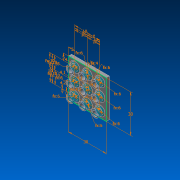
# Autodesk Inventor part: collet test
Saved by Autodesk Inventor 2015 (Build 190159000, 159)
## iProperties
Created: 2017-03-17
Part Number: collet test
Material: Generic
Document SubType Name: Modeling
Designer: ZigZagJoe
Density: 1 g/cm^3
Appearance: Default
Author: ZigZagJoe
Autodesk Inventor part; units mm, degrees
ref_plane "YZ Plane" through (0, 0, 0) normal (1, 0, 0) x (0, 1, 0)
ref_plane "XZ Plane" through (0, 0, 0) normal (0, 1, 0) x (-1, 0, 0)
ref_plane "XY Plane" through (0, 0, 0) normal (0, 0, 1) x (1, 0, 0)
sketch "Sketch1" plane through (0, 0, 0) normal (0, 1, 0) x (-1, 0, 0)
  line L0 (9.1164, 12.0254) -> (-20.8836, 12.0254)
  line L1 (-20.8836, 12.0254) -> (-20.8836, -17.9746)
  line L2 (-20.8836, -17.9746) -> (9.1164, -17.9746)
  line L3 (9.1164, -17.9746) -> (9.1164, 12.0254)
  circle A0 centre (4.1164, 7.0254) radius 3
  circle A1 centre (4.1164, -2.9746) radius 3
  circle A2 centre (4.1164, -12.9746) radius 3
  circle A3 centre (-5.8836, 7.0254) radius 3
  circle A4 centre (-5.8836, -2.9746) radius 3
  circle A5 centre (-5.8836, -12.9746) radius 3
  circle A6 centre (-15.8836, 7.0254) radius 3
  circle A7 centre (-15.8836, -2.9746) radius 3
  circle A8 centre (-15.8836, -12.9746) radius 3
  circle A9 centre (4.1164, 7.0254) radius 2
  circle A10 centre (4.1164, -2.9746) radius 2.05
  circle A11 centre (4.1164, -12.9746) radius 2.1
  circle A12 centre (-5.8836, 7.0254) radius 2
  circle A13 centre (-5.8836, -2.9746) radius 2.05
  circle A14 centre (-5.8836, -12.9746) radius 2.1
  circle A15 centre (-15.8836, 7.0254) radius 2
  circle A16 centre (-15.8836, -2.9746) radius 2.05
  circle A17 centre (-15.8836, -12.9746) radius 2.1
  line L4 (9.1164, -14.3717) -> (4.1164, -17.9746)
  point P0 (0, 0)
  dimension "d0" = 30
  dimension "d1" = 30
  dimension "d2" = 6
  dimension "d3" = 6
  dimension "d5" = 6
  dimension "d6" = 6
  dimension "d8" = 6
  dimension "d9" = 6
  dimension "d11" = 10
  dimension "d12" = 10
  dimension "d13" = 10
  dimension "d14" = 10
  dimension "d15" = 10
  dimension "d16" = 10
  dimension "d17" = 0
  dimension "d18" = 0
  dimension "d19" = 5
  dimension "d20" = 5
  dimension "d21" = 10
  dimension "d22" = 10
  dimension "d23" = 10
  dimension "d24" = 10
  dimension "d25" = 10
  dimension "d26" = 10
  dimension "d27" = 6
  dimension "d28" = 6
  dimension "d29" = 4
  dimension "d30" = 6
  dimension "d31" = 4.1
  dimension "d32" = 4.2
  dimension "d33" = 4
  dimension "d34" = 4.1
  dimension "d35" = 4.2
  dimension "d36" = 4
  dimension "d37" = 4.1
  dimension "d38" = 4.2
  constraints: 18 centre point, 10 end point, 9 coincident, 2 parallel, 2 point on line, 1 horizontal, 1 perpendicular
  measures "d0" distance of L2.end L1.end
  measures "d1" distance of L0.end L1.end
  measures "d2" diameter of A0
  measures "d3" diameter of A1
  measures "d5" diameter of A3
  measures "d6" diameter of A4
  measures "d8" diameter of A6
  measures "d9" diameter of A7
  measures "d11" distance of A1.centre A2.centre
  measures "d12" distance of A1.centre A0.centre
  measures "d13" distance of A4.centre A3.centre
  measures "d14" distance of A4.centre A5.centre
  measures "d15" distance of A7.centre A8.centre
  measures "d16" distance of A7.centre A6.centre
  measures "d17" vertical distance of A5.centre A2.centre
  measures "d18" vertical distance of A5.centre A8.centre
  measures "d19" distance from line of L0 A0.centre
  measures "d20" distance from line of L3 A0.centre
  measures "d21" distance of A3.centre A0.centre
  measures "d22" distance of A6.centre A3.centre
  measures "d23" distance of A7.centre A4.centre
  measures "d24" distance of A8.centre A5.centre
  measures "d25" distance of A5.centre A2.centre
  measures "d26" distance of A4.centre A1.centre
  measures "d27" diameter of A5
  measures "d28" diameter of A8
  measures "d29" diameter of A9
  measures "d30" diameter of A2
  measures "d31" diameter of A10
  measures "d32" diameter of A11
  measures "d33" diameter of A12
  measures "d34" diameter of A13
  measures "d35" diameter of A14
  measures "d36" diameter of A15
  measures "d37" diameter of A16
  measures "d38" diameter of A17
extrude "Extrusion1" add sketch "Sketch1" along normal blind 2.5 contours L3 L4 L2 L1 L0 | L3 L2 L4 | A0 | A1 | A2 | A3 | A4 | A5 | A6 | A7 | A8 | A9 | A10 | A11 | A12 | A13 | A14 | A15 | A16 | A17
extrude "Extrusion2" add sketch "Sketch1" against normal blind 4 contours A0 | A1 | A2 | A3 | A4 | A5 | A6 | A7 | A8
fillet "Fillet1" radius 1 9 edges at (-1.1164, 0, 7.0254) (-1.1164, 0, -2.9746) (-1.1164, 0, -12.9746) (8.8836, 0, -12.9746) (8.8836, 0, -2.9746) (8.8836, 0, 7.0254) (18.8836, 0, 7.0254) (18.8836, 0, -2.9746) (18.8836, 0, -12.9746)
extrude "Extrusion4" cut sketch "Sketch1" along normal blind 2 contours L3 L2 L4
equation "\"d3\" = d2"
equation "\"d5\" = d2"
equation "\"d6\" = d2"
equation "\"d8\" = d2"
equation "\"d9\" = d2"
equation "\"d12\" = d11"
equation "\"d13\" = d12"
equation "\"d14\" = d11"
equation "\"d15\" = d14"
equation "\"d16\" = d15"
equation "\"d27\" = d2"
equation "\"d28\" = d2"
equation "\"d30\" = d2"
equation "\"d33\" = d29"
equation "\"d34\" = d31"
equation "\"d35\" = d32"
equation "\"d36\" = d29"
equation "\"d37\" = d31"
equation "\"d38\" = d32"
body "Solid1"
